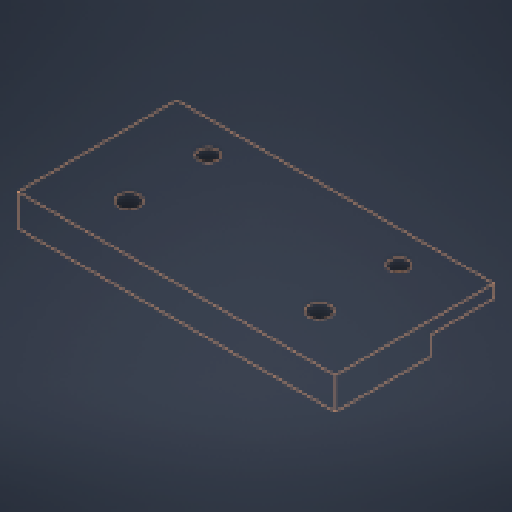
# Autodesk Inventor part: Beam Cover Bracket
Saved by Autodesk Inventor 2023.1 (Build 271208000, 208)
## iProperties
Created: 2023-02-24
Part Number: Beam Cover Bracket
Material: ABS Plastic
Document SubType Name: Modeling
Designer: remop
Density: 1.06 g/cm^3
Appearance: Smooth - Light Orange
Author: remop
Autodesk Inventor part; units mm, degrees
ref_plane "YZ Plane" through (0, 0, 0) normal (1, 0, 0) x (0, 1, 0)
ref_plane "XZ Plane" through (0, 0, 0) normal (0, 1, 0) x (-1, 0, 0)
ref_plane "XY Plane" through (0, 0, 0) normal (0, 0, 1) x (1, 0, 0)
sketch "Sketch13" plane through (0, 0, 0) normal (0, 0, 1) x (1, 0, 0)
  line L0 (-25, 12.5) -> (25, 12.5)
  line L1 (25, 12.5) -> (25, -12.5)
  line L2 (25, -12.5) -> (-25, -12.5)
  line L3 (-25, -12.5) -> (-25, 12.5)
  line L4 (-25, 12.5) -> (25, -12.5) construction
  line L5 (25, 12.5) -> (-25, -12.5) construction
  point P0 (0, 0)
  dimension "d26" = 50
  dimension "d27" = 25
  constraints: 12 end point, 2 midpoint, 2 parallel, 1 horizontal, 1 perpendicular
  measures "d26" distance of L1.end L2.end
  measures "d27" distance of L0.end L1.end
extrude "Extrusion14" add sketch "Sketch13" along normal blind 5
sketch "Sketch14" plane through (0, 0, 0) normal (0, 0, -1) x (-1, 0, 0)
  line L0 (25, -12.5) -> (-25, -12.5) projected
  line L1 (25, 12.5) -> (25, -12.5) projected
  line L2 (-25, 12.5) -> (25, 12.5) projected
  line L3 (-25, -12.5) -> (-25, 12.5) projected
  line L4 (-25, -12.5) -> (-25, 12.5) projected
  line L5 (-25, 2.5) -> (25, 2.5)
  line L6 (25, 12.5) -> (25, -12.5) projected
  point P0 (0, 0)
  point P1 (25, 2.5)
  dimension "d30" = 10
  constraints: 2 end point, 2 point on line, 1 horizontal
  measures "d30" distance between parallel lines of L2 L5
extrude "Extrusion15" cut sketch "Sketch14" against normal blind 3 contours L5 L3 L2 L1
sketch "Sketch16" plane through (0, 0, 3) normal (0, 0, -1) x (-1, 0, 0)
  line L0 (-25, 2.5) -> (-25, 12.5) projected
  line L1 (25, 2.5) -> (-25, 2.5) projected
  line L2 (25, 12.5) -> (25, 2.5) projected
  line L3 (-25, 12.5) -> (25, 12.5) projected
  point P0 (0, 0)
  point P1 (-15, 7.5)
  point P2 (15, 7.5)
  point P3 (-25, 7.5)
  point P4 (25, 7.5)
  dimension "d33" = 10
  dimension "d34" = 10
  constraints: 2 horizontal alignment, 2 midpoint
  measures "d33" distance from line of L0 point (-15, 7.5)
  measures "d34" distance from line of L2 point (15, 7.5)
hole "Hole1" at (15, 7.5, 3) at (-15, 7.5, 3) direction (0, 0, 1) diameter 2.9 end through all
sketch "Sketch17" plane through (0, 0, 5) normal (0, 0, 1) x (1, 0, 0)
  line L0 (-25, 12.5) -> (-25, -12.5) projected
  line L1 (25, -12.5) -> (25, 12.5) projected
  point P0 (0, 0)
  point P1 (-15, -5)
  point P2 (15, -5)
  dimension "d42" = 7.5
  dimension "d43" = 10
  dimension "d44" = 10
  constraints: 1 horizontal alignment
  measures "d42" vertical distance of L0.end point (-15, -5)
  measures "d43" distance from line of L1 point (15, -5)
  measures "d44" distance from line of L0 point (-15, -5)
hole "Hole2" at (-15, -5, 5) at (15, -5, 5) direction (0, 0, -1) diameter 3.2 end through all
equation "\"d34\" = d33"
equation "\"d44\" = d43"
body "Solid11"
